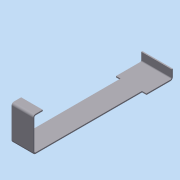
# Autodesk Inventor part: Umbilicals_Tape_USB
Saved by Autodesk Inventor 2014 SP1 (Build 180222100, 222)
## iProperties
Created: 2013-03-20
Material: Aluminum-6061
Document SubType Name: Sheet Metal
Designer: Robert Davis
Mass: 0.172085 g
Surface Area: 2.767 cm^2
Volume: 0.0635 cm^3
Density: 2.71 g/cm^3
Description: 1ST SURF METAL TAPE
Appearance: Aluminum - Flat
Sheet Metal Rule: Default
Part Number: Umbilicals_Tape_USB
Author: Robert Davis
Autodesk Inventor part; units mm, degrees
ref_plane "YZ Plane" through (0, 0, 0) normal (1, 0, 0) x (0, 1, 0)
ref_plane "XZ Plane" through (0, 0, 0) normal (0, 1, 0) x (-1, 0, 0)
ref_plane "XY Plane" through (0, 0, 0) normal (0, 0, 1) x (1, 0, 0)
sketch "Sketch1" plane through (0, 0, 0) normal (0, 0, 1) x (1, 0, 0)
  line L0 (0, 0) -> (6.3089, 0)
  line L1 (0, 0) -> (0, 8.1845)
  line L2 (4.5, 24) -> (4.5, -35)
  line L3 (4.5, -35) -> (-4.5, -35)
  line L4 (-4.5, -35) -> (-4.5, 24)
  line L5 (-6.35, 35) -> (6.35, 35)
  line L6 (6.35, 35) -> (6.35, 24)
  line L7 (-6.35, 24) -> (-6.35, 35)
  line L8 (6.35, 24) -> (4.5, 24)
  line L9 (-4.5, 24) -> (-6.35, 24)
  dimension "d4" = 9
  dimension "d5" = 12.7
  dimension "d6" = 70
  dimension "d7" = 11
  constraints: 20 end point, 4 parallel, 3 horizontal, 3 vertical, 1 coincident, 1 perpendicular, 3 other
  measures "d4" distance of L2.end L3.end
  measures "d5" distance of L5.start L5.end
  measures "d6" distance between parallel lines of L3 L5
  measures "d7" distance of L5.end L6.end
extrude "Extrusion1" add sketch "Sketch1" along normal blind 0.5
sketch "Sketch2" plane through (-6.35, 34.5, 0) normal (0, 1, 0) x (-1, 0, 0)
  line L0 (-12.7, 0) -> (0, 0)
  line L1 (0, 0) -> (0, 4)
  line L2 (0, 4) -> (-12.7, 4)
  line L3 (-12.7, 4) -> (-12.7, 0)
  constraints: 6 end point, 1 horizontal, 1 perpendicular, 1 vertical
edge flange "Flange1" height 4 angle 90 thickness 0.5 bend radius 0.5 thickness toward (0, 1, 0) relief straight relief width 0.5 relief depth 0.25 edges at (0, 35, 0.5) wall of the first edge with corners at (6.35, 34.5, 0) (-6.35, 34.5, 0) (-6.35, 34.5, 4) (6.35, 34.5, 4)
bend "Bend1"
corner "Corner1"
sketch "Sketch4" plane through (4.5, -34.5, 0) normal (0, -1, 0) x (1, 0, 0)
  line L0 (-9, 0) -> (0, 0)
  line L1 (0, 0) -> (0, 4)
  line L2 (0, 4) -> (-9, 4)
  line L3 (-9, 4) -> (-9, 0)
  constraints: 6 end point, 1 horizontal, 1 perpendicular, 1 vertical
edge flange "Flange3" height 4 angle 90 thickness 0.5 bend radius 0.5 thickness toward (0, -1, 0) relief straight relief width 0.5 relief depth 0.25 edges at (0, -35, 0.5) wall of the first edge with corners at (-4.5, -34.5, 0) (4.5, -34.5, 0) (4.5, -34.5, 4) (-4.5, -34.5, 4)
bend "Bend3"
corner "Corner3"
sketch "Sketch5" plane through (0, 0, 0.5) normal (0, 0, 1) x (1, 0, 0)
  line L0 (4.5, 24) -> (4.5, -34) projected
  line L1 (6.35, 24) -> (4.5, 24) projected
  line L2 (-4.5, -34) -> (-4.5, 24) projected
  line L3 (-4.5, -21) -> (4.5, -21)
  point P0 (0, 0)
  dimension "d38" = 45
  constraints: 2 end point, 2 point on line, 1 horizontal
  measures "d38" distance between parallel lines of L1 L3
fold "Fold1" angle 90 bend radius 0.5 thickness 0.5 k factor 0.44 line from (-4.5, -21, 0.5) to (4.5, -21, 0.5) line at bend centre moving side (0, -1, 0) folds toward (0, 0, 1)
equation "\"d39\" = BendReliefWidth"
equation "\"d40\" = BendReliefDepth"
equation "\"d41\" = MinimumRemnant"
equation "\"d42\" = BendRadius"
equation "\"d44\" = BendRadius"
equation "\"d8\" = BendReliefWidth"
equation "\"d9\" = BendReliefDepth"
equation "\"d10\" = MinimumRemnant"
equation "\"d11\" = BendRadius"
equation "\"d14\" = BendRadius"
equation "\"d15\" = CornerReliefSize"
equation "\"d16\" = GapSize"
equation "\"d17\" = JacobiRadiusSize"
equation "\"d28\" = BendReliefWidth"
equation "\"d29\" = BendReliefDepth"
equation "\"d30\" = MinimumRemnant"
equation "\"d31\" = BendRadius"
equation "\"d34\" = BendRadius"
equation "\"d35\" = CornerReliefSize"
equation "\"d36\" = GapSize"
equation "\"d37\" = JacobiRadiusSize"
equation "\"BendRadius\" = Thickness"
equation "\"BendReliefWidth\" = Thickness"
equation "\"BendReliefDepth\" = 0.5 * Thickness"
equation "\"CornerReliefSize\" = 4 * Thickness"
equation "\"MinimumRemnant\" = 2 * Thickness"
equation "\"TransitionRadius\" = BendRadius"
equation "\"JacobiRadiusSize\" = Thickness"
equation "\"GapSize\" = Thickness"
equation "\"Thickness\" = 0.5"
body "Solid1"
